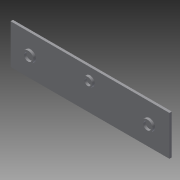
# Autodesk Inventor part: z rods top bracket
Saved by Autodesk Inventor 2014 SP1 (Build 180222100, 222)
## iProperties
Created: 2014-10-11
Part Number: z rods top bracket
Material: Generic
Document SubType Name: Modeling
Designer: Mon
Density: 1 g/cm^3
Appearance: Default
Author: Mon
Autodesk Inventor part; units mm, degrees
ref_plane "YZ Plane" through (0, 0, 0) normal (1, 0, 0) x (0, 1, 0)
ref_plane "XZ Plane" through (0, 0, 0) normal (0, 1, 0) x (-1, 0, 0)
ref_plane "XY Plane" through (0, 0, 0) normal (0, 0, 1) x (1, 0, 0)
sketch "Sketch1" plane through (0, 0, 0) normal (0, 1, 0) x (-1, 0, 0)
  line L0 (0, 0) -> (200, 0)
  line L1 (200, 0) -> (200, 50)
  line L2 (200, 50) -> (0, 50)
  line L3 (0, 50) -> (0, 0)
  line L4 (100, 50) -> (100, -12.2978) construction
  line L5 (100, 46.202) -> (25, 46.202) construction
  line L6 (25, 46.202) -> (25, 4.511) construction
  line L7 (14.6583, 50) -> (14.6583, 25) construction
  line L8 (14.6583, 25) -> (197.0399, 25) construction
  line L9 (110.8785, 50) -> (110.8785, 35) construction
  line L10 (110.8785, 35) -> (88.7756, 35) construction
  dimension "d0" = 200
  dimension "d1" = 50
  dimension "d2" = 75
  dimension "d3" = 25
  dimension "d4" = 15
  constraints: 22 end point, 6 perpendicular, 4 parallel, 3 point on line, 1 horizontal, 1 midpoint
  measures "d0" distance of L2.end L1.end
  measures "d1" distance of L1.end L0.end
  measures "d2" distance of L5.start L5.end
  measures "d3" distance of L7.start L7.end
  measures "d4" distance of L9.start L9.end
extrude "Extrusion1" add sketch "Sketch1" along normal blind 3
sketch "Sketch2" plane through (0, 0, 0) normal (0, -1, 0) x (1, 0, 0)
  line L0 (0, 0) -> (-200, 0) projected
  line L1 (-200, 50) -> (0, 50) projected
  line L2 (-200, 0) -> (-200, 50) projected
  line L3 (-100, 50) -> (-100, -20.2581) construction
  line L4 (-200, 25) -> (-5.0979, 25) construction
  line L5 (-100, 50) -> (-100, 35) construction
  line L6 (-100, 35) -> (-80.8703, 35) construction
  line L7 (-100, 35) -> (-119.3164, 35) construction
  line L8 (-190.2363, 50) -> (-190.2363, 25) construction
  line L9 (-100, 0) -> (-175, 0) construction
  line L10 (-175, 0) -> (-175, 41.5169) construction
  line L11 (-100, 0) -> (-25, 0) construction
  line L12 (-25, 0) -> (-25, 41.5169) construction
  circle A0 centre (-100, 35) radius 4
  circle A1 centre (-100, 35) radius 6
  dimension "d7" = 15
  dimension "d8" = 25
  dimension "d9" = 75
  dimension "d10" = 75
  dimension "d11" = 8
  dimension "d12" = 12
  constraints: 20 end point, 6 point on line, 4 perpendicular, 3 midpoint, 2 centre point, 2 coincident, 1 collinear, 1 parallel
  measures "d7" distance of L3.start L5.end
  measures "d8" distance of L8.start L8.end
  measures "d9" distance of L9.start L9.end
  measures "d10" distance of L9.start L11.end
  measures "d11" diameter of A0
  measures "d12" diameter of A1
extrude "Extrusion2" add sketch "Sketch2" along normal blind 3
sketch "Sketch3" plane through (0, 0, 0) normal (0, -1, 0) x (1, 0, 0)
  line L0 (-200, 50) -> (0, 50) projected
  line L1 (-200, 0) -> (-200, 50) projected
  circle A0 centre (-100, 35) radius 6 projected
  line L2 (-100, 35) -> (-175, 35) construction
  line L3 (-175, 35) -> (-175, -16.3605) construction
  line L4 (-191.9526, 50) -> (-191.9526, 25) construction
  line L5 (-191.9526, 25) -> (-42.7931, 25) construction
  circle A1 centre (-175, 25) radius 5
  circle A2 centre (-175, 25) radius 7
  dimension "d15" = 75
  dimension "d16" = 25
  dimension "d17" = 10
  dimension "d18" = 14
  constraints: 8 end point, 3 perpendicular, 3 point on line, 2 centre point, 1 coincident, 1 parallel
  measures "d15" distance of L2.start L2.end
  measures "d16" distance of L4.start L4.end
  measures "d17" diameter of A1
  measures "d18" diameter of A2
extrude "Extrusion3" add sketch "Sketch3" along normal blind 3 contours A2
sketch "Sketch4" plane through (0, 0, 0) normal (0, -1, 0) x (1, 0, 0)
  circle A0 centre (-100, 35) radius 6 projected
  line L0 (-200, 50) -> (0, 50) projected
  line L1 (-200, 0) -> (-200, 50) projected
  line L2 (-100, 35) -> (-25, 35) construction
  line L3 (-25, 35) -> (-25, -20.2088) construction
  line L4 (-14.8647, 50) -> (-14.8647, 25) construction
  line L5 (-14.8647, 25) -> (-71.3929, 25) construction
  circle A1 centre (-25, 25) radius 5
  circle A2 centre (-25, 25) radius 7
  dimension "d21" = 75
  dimension "d22" = 25
  dimension "d23" = 10
  dimension "d24" = 14
  constraints: 8 end point, 3 perpendicular, 3 point on line, 2 centre point, 1 coincident, 1 parallel
  measures "d21" distance of L2.start L2.end
  measures "d22" distance of L4.start L4.end
  measures "d23" diameter of A1
  measures "d24" diameter of A2
extrude "Extrusion4" add sketch "Sketch4" along normal blind 3 contours A2
body "Solid1"
